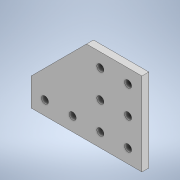
# Autodesk Inventor part: 2x1 L plate
Saved by Autodesk Inventor 2020 (Build 240168000, 168)
## iProperties
Created: 2020-01-14
Part Number: 2x1 L plate
Material: Generic
Document SubType Name: Modeling
Designer: 329817
Density: 1 g/cm^3
Appearance: Default
Author: 329817
Autodesk Inventor part; units mm, degrees
ref_plane "YZ Plane" through (0, 0, 0) normal (1, 0, 0) x (0, 1, 0)
ref_plane "XZ Plane" through (0, 0, 0) normal (0, 1, 0) x (-1, 0, 0)
ref_plane "XY Plane" through (0, 0, 0) normal (0, 0, 1) x (1, 0, 0)
sketch "Sketch1" plane through (0, 0, 0) normal (0, 0, 1) x (1, 0, 0)
  line L0 (0, 0) -> (101.6, 0)
  line L1 (101.6, 0) -> (101.6, 76.2)
  line L2 (101.6, 76.2) -> (50.8, 76.2)
  line L3 (0, 25.4) -> (0, 0)
  circle A0 centre (12.7, 12.7) radius 3.2512
  circle A1 centre (38.1, 12.7) radius 3.2512
  circle A2 centre (63.5, 12.7) radius 3.2512
  circle A3 centre (88.9, 12.7) radius 3.2512
  line L4 (101.6, 25.4) -> (101.6, 101.6)
  circle A4 centre (88.9, 38.1) radius 3.2512
  circle A5 centre (63.5, 38.1) radius 3.2512
  line L5 (101.6, 50.8) -> (101.6, 127)
  circle A6 centre (88.9, 63.5) radius 3.2512
  circle A7 centre (63.5, 63.5) radius 3.2512
  line L6 (50.8, 76.2) -> (0, 25.4)
  dimension "d0" = 101.6
  dimension "d1" = 76.2
  dimension "d2" = 25.4
  dimension "d3" = 6.5024
  dimension "d4" = 12.7
  dimension "d5" = 12.7
  dimension "d8" = 25.4
  dimension "d15" = 25.4
  dimension "d20" = 50.8
  constraints: 14 end point, 8 centre point, 2 horizontal, 2 parallel, 1 coincident, 1 collinear, 1 perpendicular, 1 vertical, 19 other
  measures "d0" distance of L0.start L0.end
  measures "d1" distance of L0.end L1.end
  measures "d2" distance of L3.start L0.start
  measures "d3" diameter of A0
  measures "d4" distance from line of L0 A0.centre
  measures "d5" distance from line of L3 A0.centre
  measures "d8" distance of A0.centre A1.centre
  measures "d15" distance of L0.end L4.start
  measures "d20" distance of L2.end L1.end
extrude "Extrusion1" add sketch "Sketch1" along normal blind 6.35
body "Solid1"
